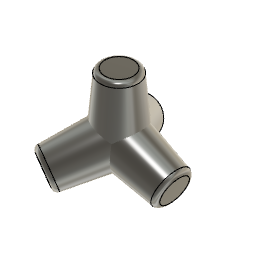
tetrapod v1 (Autodesk Fusion 360 design; units mm, degrees)
Autodesk Fusion 360 part; units mm, degrees
sketch "スケッチ1" plane through (0, 0, 0) normal (0, 0, 1) x (1, 0, 0)
  circle A0 centre (0, 0) radius 20
  dimension "d1" = 40
  constraint coincident A0.centre origin
  measures "d1" diameter of A0
extrude "押し出し1" add sketch "スケッチ1" along normal blind 50 draft -5 makes body 1
fillet "フィレット1" radius 4 1 edges at (-14.5681, 5.6504, 50) on bodies 1
copy_body "ボディのコピーと貼り付け1" bodies 1 makes body 2
move_body "移動1" bodies 2 to x (-0.33333, 0, -0.94281) y (0, 1, 0) z (0.94281, 0, -0.33333) at (0, 0, 0)
pattern_circular "C パターン1" count 3 over 360 about axis through (0, 0, 0) along (0, 0, 1) of bodies 2 makes body 3 at (10.9267, 7.5458, -15.5088) makes body 4 at (-19.7854, 1.959, 4.6428)
